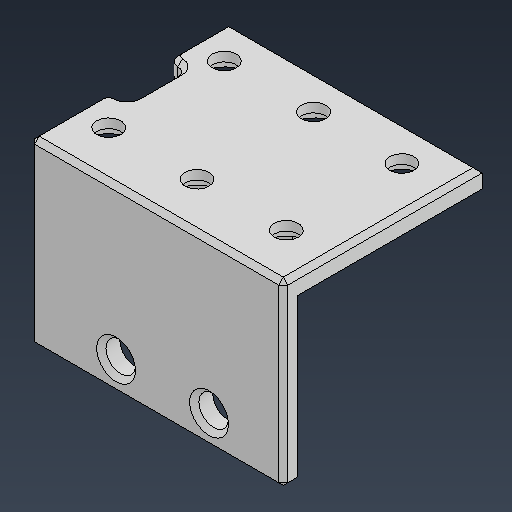
# Autodesk Inventor part: BackLunaRecoveryHold
Saved by Autodesk Inventor 2026.2 (Build 302298010, 298A)
## iProperties
Created: 2026-07-04
Part Number: BackLunaRecoveryHold
Material: Generic
Document SubType Name: Modeling
Designer: szymo
Density: 1 g/cm^3
Appearance: Default
Author: szymo
Autodesk Inventor part; units mm, degrees
ref_plane "YZ Plane" through (0, 0, 0) normal (1, 0, 0) x (0, 1, 0)
ref_plane "XZ Plane" through (0, 0, 0) normal (0, 1, 0) x (-1, 0, 0)
ref_plane "XY Plane" through (0, 0, 0) normal (0, 0, 1) x (1, 0, 0)
sketch "Sketch1" plane through (0, 0, 0) normal (1, 0, 0) x (0, 1, 0)
  line L0 (-60.9278, 7.9432) -> (-60.9278, 6.9432)
  line L1 (-60.9278, 6.9432) -> (-53.2278, 6.9432)
  line L2 (-53.2278, 7.9432) -> (-53.2278, 6.9432)
  line L3 (-60.9278, 7.9432) -> (-53.2278, 7.9432)
  line L4 (-70.2278, 7.9432) -> (-70.2278, 6.9432)
  line L5 (-70.2278, 6.9432) -> (-60.9278, 6.9432)
  line L6 (-60.9278, 6.9432) -> (-60.9278, 7.9432)
  line L7 (-70.2278, 7.9432) -> (-60.9278, 7.9432)
  line L8 (-53.2278, 6.9432) -> (-53.2278, 5.4432)
  line L9 (-53.2278, 5.4432) -> (-53.2278, 1.4432)
  line L10 (-53.2278, -5.0568) -> (-53.2278, -9.0568)
  line L11 (-53.2278, -9.0568) -> (-53.2278, -9.5568)
  line L12 (-53.2278, -9.5568) -> (-53.2278, -11.5568)
  line L13 (-70.2278, 7.9432) -> (-53.2278, 7.9432)
  line L14 (-53.2278, 7.9432) -> (-53.2278, -11.5568)
  line L15 (-53.2278, -11.5568) -> (-50.7278, -11.5568)
  line L16 (-39.4278, 9.9432) -> (-70.2278, 9.9432)
  line L17 (-70.2278, 9.9432) -> (-70.2278, 7.9432)
  line L18 (-39.4278, 9.9432) -> (-39.4278, 7.9432)
  line L19 (-39.4278, 7.9432) -> (-50.7278, 7.9432)
  line L20 (-50.7278, 7.9432) -> (-50.7278, -11.5568)
  line L21 (-50.7278, 7.9432) -> (-50.7278, 9.9432)
  point P0 (0, 0)
extrude "Extrusion1" add sketch "Sketch1" against normal blind 27.4 contours L7 L17 L16 L21 L20 L15 L12 L11 L10 L14 L9 L8 L2 L3
sketch "Sketch2" plane through (0, -53.2278, -11.5568) normal (0, -1, 0) x (1, 0, 0)
  circle A0 centre (-4.725, 16.4491) radius 0.7835 projected
  circle A1 centre (-14.325, 16.5) radius 0.7835 projected
  circle A2 centre (-23.925, 16.4491) radius 0.7835 projected
  circle A3 centre (-4.725, 3.9509) radius 0.7835 construction
  circle A4 centre (-14.325, 3.9) radius 0.7835 construction
  circle A5 centre (-23.925, 3.9509) radius 0.7835 construction
  line L0 (-6.5, 13) -> (-27.4, 13) projected
  line L1 (-27.4, 6.5) -> (-6.5, 6.5) projected
  line L2 (-29.4, 13) -> (-25.4, 13)
  line L3 (-25.4, 13) -> (-25.4, 6.5)
  line L4 (-25.4, 6.5) -> (-29.4, 6.5)
  line L5 (-29.4, 6.5) -> (-29.4, 13)
  point P0 (0, 11.5568)
  dimension "d6" = 2
  dimension "d7" = 2
  constraints: 8 end point, 2 parallel, 2 point on line, 1 horizontal, 1 perpendicular
  measures "d6" distance from line of L5 L0.end
  measures "d7" distance from line of L1.start L3
hole "Hole1" at (-23.925, -53.2278, 4.8923) at (-4.725, -53.2278, 4.8923) at (-14.325, -53.2278, 4.9432) at (-4.725, -53.2278, -7.6059) at (-14.325, -53.2278, -7.6568) at (-23.925, -53.2278, -7.6059) direction (0, 1, 0) diameter 2.6 depth 11.5 counterbore diameter 5.5 counterbore depth 1.5 clearance for "Countersunk Flat Head Screw ISO 2009/7046" size "M2" standard "ISO"
sketch "Sketch3" plane through (0, -50.7278, 7.9432) normal (0, 1, 0) x (1, 0, 0)
  line L0 (-6.5, 6.5) -> (-27.4, 6.5) projected
  line L1 (-27.4, 13) -> (-6.5, 13) projected
  line L2 (-29.4, 6.5) -> (-25.4, 6.5)
  line L3 (-25.4, 6.5) -> (-25.4, 13)
  line L4 (-25.4, 13) -> (-29.4, 13)
  line L5 (-29.4, 13) -> (-29.4, 6.5)
  point P0 (0, 7.9432)
  dimension "d15" = 2
  dimension "d16" = 2
  constraints: 8 end point, 2 midpoint, 2 parallel, 1 horizontal, 1 perpendicular
  measures "d15" distance from line of L5 L0.end
  measures "d16" distance from line of L0.end L3
extrude "Extrusion2" cut sketch "Sketch3" against normal blind 27.4
fillet "Fillet1" radius 1 4 edges at (-25.4, -51.9778, 1.4432) (-25.4, -51.9778, -5.0568) (-27.4, -51.9778, -5.0568) (-27.4, -51.9778, 1.4432)
sketch "Sketch4" plane through (0, -70.2278, 9.9432) normal (0, 0, 1) x (1, 0, 0)
  circle A0 centre (-8.025, 3.25) radius 1.2295 projected
  circle A1 centre (-18.075, 3.25) radius 1.2295 projected
  point P0 (0, 70.2278)
hole "Hole2" at (-18.075, -66.9778, 9.9432) at (-8.025, -66.9778, 9.9432) direction (0, 0, -1) diameter 3.2 depth 10 clearance for "Countersunk Flat Head Screw ISO 2009/7046" size "M3" standard "ISO"
chamfer "Chamfer1" distance 0.5 angle 45 2 edges at (-18.075, -65.3778, 9.9432) (-8.025, -65.3778, 9.9432)
sketch "Sketch5" plane through (0, -53.2278, -11.5568) normal (0, -1, 0) x (1, 0, 0)
  line L0 (-27.4, 6.5) -> (-6.5, 6.5) projected
  line L1 (-6.5, 13) -> (-27.4, 13) projected
  line L2 (-6.5, 6.5) -> (-6.5, 13)
  line L3 (-25.4, 6.5) -> (-25.4, 13)
  point P0 (0, 11.5568)
  dimension "d30" = 2
  constraints: 4 end point, 2 point on line, 1 perpendicular, 1 vertical
  measures "d30" distance from line of L3 L0.start
extrude "Extrusion3" add sketch "Sketch5" along normal blind 3.7
chamfer "Chamfer2" distance 1 angle 45 2 edges at (-15.95, -56.9278, -5.0568) (-15.95, -56.9278, 1.4432)
fillet "Fillet2" radius 1 14 edges at (-15.95, -55.9278, -5.0568) (-15.95, -56.9278, -4.0568) (-15.95, -56.9278, 0.4432) (-15.95, -55.9278, 1.4432) (-6.5, -54.5778, -5.0568) (-6.5, -56.4278, -4.5568) (-6.5, -56.9278, -1.8068) (-6.5, -56.4278, 0.9432) (-6.5, -54.5778, 1.4432) (-25.4, -54.5778, -5.0568) (-25.4, -56.4278, -4.5568) (-25.4, -56.9278, -1.8068) (-25.4, -56.4278, 0.9432) (-25.4, -54.5778, 1.4432)
chamfer "Chamfer3" distance 0.5 angle 45 29 edges at (-27.4, -50.7278, 6.1932) (-26.4, -50.7278, 1.4432) (-27.1071, -50.7278, 1.7361) (-25.6929, -50.7278, 1.1504) (-25.4, -50.7278, -1.8068) (-26.4, -50.7278, -5.0568) (-25.6929, -50.7278, -4.7639) (-27.1071, -50.7278, -5.3496) (-27.4, -50.7278, -8.8067) (-13.7, -50.7278, -11.5568) (0, -50.7278, -0.8068) (-13.7, -50.7278, 9.9432) (-13.7, -53.2278, -11.5568) (0, -53.2278, -1.8068) (0, -61.7278, 7.9432) (0, -60.4778, 9.9432) (0, -70.2278, 8.9432) (-13.7, -70.2278, 9.9432) (-27.4, -60.4778, 9.9432) (-13.7, -70.2278, 7.9432) (-27.4, -61.7278, 7.9432) (-27.4, -53.2278, 5.1932) (-27.1071, -53.2278, 1.7361) (-26.4, -53.2278, 1.4432) (-25.6929, -53.2278, 1.1504) (-27.4, -53.2278, -8.8067) (-27.1071, -53.2278, -5.3496) (-26.4, -53.2278, -5.0568) (-25.6929, -53.2278, -4.7639)
body "Solid1"
